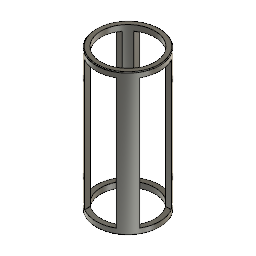
Pre+Filter (Autodesk Fusion 360 design; units mm, degrees)
Autodesk Fusion 360 part; units mm, degrees
sketch "Sketch1" plane through (0, 0, 0) normal (0, 0, 1) x (1, 0, 0)
  circle A0 centre (0, 0) radius 22.5
  circle A1 centre (0, 0) radius 19
  dimension "d1" = 45
  dimension "d2" = 38
  constraint coincident A0.centre A1.centre
  measures "d1" diameter of A0
  measures "d2" diameter of A1
extrude "Extrude1" add sketch "Sketch1" along normal blind 100
sketch "Sketch2" plane through (0, 0, 0) normal (0, 1, 0) x (1, 0, 0)
  line L0 (-3.75, -96) -> (11.25, -96)
  line L1 (11.25, -96) -> (11.25, -4)
  line L2 (11.25, -4) -> (-3.75, -4)
  line L3 (-3.75, -4) -> (-3.75, -96)
  line L4 (-22.5, -100) -> (22.5, -100)
  line L5 (-22.5, 0) -> (22.5, 0)
  line L6 (0, -120) -> (0, 0)
  dimension "d5" = 4
  dimension "d7" = 4
  dimension "d8" = 15
  constraint horizontal L0
  constraint vertical L1
  constraint horizontal L2
  constraint vertical L3
  constraint coincident L6.end origin
  constraint perpendicular L5 L6
  measures "d5" distance of L0 L4
  measures "d7" distance of L2 L5
  measures "d8" distance of L0.start L0.end
extrude "Extrude2" cut sketch "Sketch2" along normal blind 30 and the other way blind 40
pattern_circular "C-Pattern1" count 4 over 360 about axis through (0, 0, 1.75) along (0, 0, 1) of "Extrude2"
fillet "Fillet1" radius 0.5 1 edges at (-20.977365, -8.136347, 100)
fillet "Fillet2" radius 0.5 1 edges at (-20.977365, -8.136347, 0)
sketch "Sketch3" plane through (0, 0, 0) normal (0, 0, 1) x (1, 0, 0)
ref_plane "WorkPlane1" through (16.052642, 15.765871, 80.278568) normal (0.713451, 0.700705, 0) x (0.700705, -0.713451, 0)
sketch "Sketch4" plane through (16.052642, 15.765871, 80.278568) normal (0.713451, 0.700705, 0) x (0.700705, -0.713451, 0)
  circle A0 centre (0, 0) radius 1.7
  circle A1 centre (0, 60) radius 1.7
  dimension "d22" = 3.4
  dimension "d23" = 60
  constraint coincident A0.centre origin
  constraint equal A0 A1
  measures "d22" diameter of A0
  measures "d23" distance of A0.centre A1.centre
extrude "Extrude3" cut sketch "Sketch4" against normal blind 65
